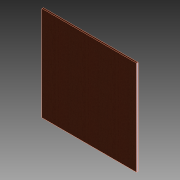
# Autodesk Inventor part: 5100_Base_Board_MPSv2_v1
Saved by Autodesk Inventor 2021 (Build 250183000, 183)
## iProperties
Created: 2021-05-17
Part Number: 5100_Base_Board_MPSv2_v1
Material: Wood (Oak)
Document SubType Name: Modeling
Designer: Barksdale
Density: 0.76 g/cm^3
Appearance: White Oak - Natural Medium Gloss
Author: Barksdale
Autodesk Inventor part; units mm, degrees
ref_plane "YZ Plane" through (0, 0, 0) normal (1, 0, 0) x (0, 1, 0)
ref_plane "XZ Plane" through (0, 0, 0) normal (0, 1, 0) x (-1, 0, 0)
ref_plane "XY Plane" through (0, 0, 0) normal (0, 0, 1) x (1, 0, 0)
sketch "Sketch1" plane through (0, 0, 0) normal (0, 0, 1) x (1, 0, 0)
  line L0 (-400, 400) -> (400, 400)
  line L1 (400, 400) -> (400, -400)
  line L2 (400, -400) -> (-400, -400)
  line L3 (-400, -400) -> (-400, 400)
  line L4 (-400, 400) -> (400, -400) construction
  line L5 (400, 400) -> (-400, -400) construction
  point P0 (0, 0)
  dimension "d0" = 800
  dimension "d1" = 800
  constraints: 12 end point, 2 midpoint, 2 parallel, 1 horizontal, 1 perpendicular
  measures "d0" distance of L1.end L2.end
  measures "d1" distance of L0.end L1.end
extrude "Extrusion1" add sketch "Sketch1" along normal blind 12.7
body "Solid1"
